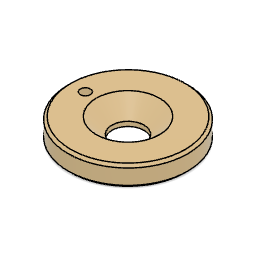
BC vertical rod endcap v5 (Autodesk Fusion 360 design; units mm, degrees)
Autodesk Fusion 360 part; units mm, degrees
note: some values were not read from the file. Set by a fixed rule: the direction of a hole.
cylinder "CylinderPrimitive1" add diameter 23.8 height 4 placed x (1, 0, 0) y (0, 0, -1) z (0, 1, 0) at (0, 0, 0)
hole "Hole1" at (0, 4, 0) direction (0, -1, 0) diameter 6.4 end through all countersink diameter 12.6 countersink angle 90
chamfer "Chamfer1" distance 0.5 angle 45 2 edges at (-11.0947, 4, 4.3032) (-11.0947, 0, -4.3032)
sketch "Sketch4" plane through (0, 0, 0) normal (0, 1, 0) x (1, 0, 0)
  circle A0 centre (0, 0) radius 8.5 construction
  point P0 (-8.5, 0)
  dimension "d9" = 17
  constraint coincident A0.centre origin
  constraint coincident A0 P0
  constraint horizontal A0.centre P0
  measures "d9" diameter of A0
hole "Hole2" at (-8.5, 0, 0) direction (0, 1, 0) diameter 2 end through all
